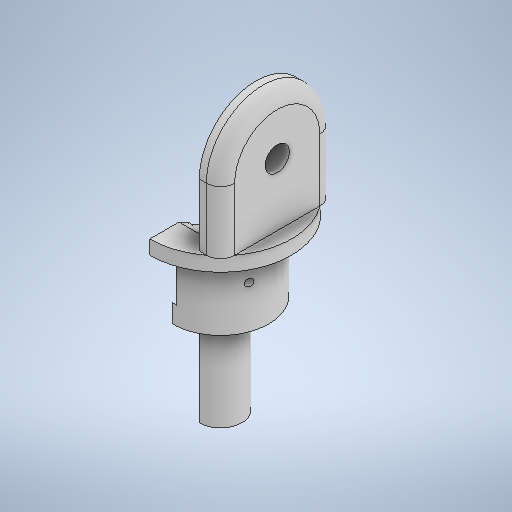
# Autodesk Inventor part: Haltevorrichtung1
Saved by Autodesk Inventor 2025 (Build 290162010, 162A)
## iProperties
Created: 2024-11-19
Part Number: Haltevorrichtung1
Material: Generisch
Document SubType Name: Modeling
Designer: jensb
Density: 1 g/cm^3
Appearance: Vorgabe
Author: jensb
Autodesk Inventor part; units mm, degrees
ref_plane "YZ Plane" through (0, 0, 0) normal (1, 0, 0) x (0, 1, 0)
ref_plane "XZ Plane" through (0, 0, 0) normal (0, 1, 0) x (-1, 0, 0)
ref_plane "XY Plane" through (0, 0, 0) normal (0, 0, 1) x (1, 0, 0)
sketch "Skizze1" plane through (0, 0, 0) normal (0, 0, 1) x (1, 0, 0)
  arc A0 (0, -15) -> (0, 15) centre (0, 0) ccw
  line L0 (0, -15) -> (0, 15)
  dimension "d27" = 15
  constraints: 2 end point, 2 point on circle, 1 centre point, 1 coincident, 1 vertical, 1 vertical alignment
  measures "d27" radius of A0
extrude "Extrusion1" add sketch "Skizze1" along normal blind 100
sketch "Skizze10" plane through (0, 0, 100) normal (0, 0, 1) x (1, 0, 0)
  arc A0 (0, -34) -> (0, 34) centre (0, 0) ccw
  line L0 (0, -34) -> (0, 34)
  dimension "d31" = 34
  constraints: 2 coincident, 2 end point, 2 point on circle, 1 centre point, 1 midpoint, 1 vertical
  measures "d31" radius of A0
extrude "Extrusion8" add sketch "Skizze10" along normal blind 20 and the other way blind 30
sketch "Skizze11" plane through (0, -15, 0) normal (-1, 0, 0) x (0, 0, 1)
  circle A0 centre (100, 3.2674) radius 25 construction
  circle A1 centre (174.0766, 15) radius 50 construction
  line L0 (174.0766, 15) -> (100, 15) construction
  line L1 (174.0766, 15) -> (100, 3.2674) construction
  circle A2 centre (100, 3.2674) radius 27.5 construction
  circle A3 centre (174.0766, 15) radius 52.5 construction
  line L2 (0, 30) -> (0, 0) construction
  line L3 (70, -19) -> (70, 0) construction
  circle A4 centre (174.0766, 15) radius 53
  point P0 (0, 15)
  point P1 (0, 15)
  dimension "d37" = 50
  dimension "d38" = 100
  dimension "d40" = 9
  dimension "d41" = 105
  dimension "d42" = 55
  dimension "d43" = 30
  dimension "d52" = 106
  dimension "d61" = 11.7326
  constraints: 5 centre point, 4 end point, 2 coincident, 1 horizontal, 1 horizontal alignment, 1 midpoint, 1 tangent, 1 vertical alignment
  measures "d37" diameter of A0
  measures "d38" diameter of A1
  measures "d40" angle of L0 L1
  measures "d41" diameter of A3
  measures "d42" diameter of A2
  measures "d43" distance from line of L3 L1.end
  measures "d52" diameter of A4
  measures "d61" distance from line of L0 L1.end
sketch "Skizze12" plane through (0, 0, 120) normal (0, 0, 1) x (1, 0, 0)
  arc A0 (0, -50) -> (0, 50) centre (0, 0) ccw
  line L0 (0, -50) -> (0, 50)
  dimension "d39" = 50
  constraints: 2 coincident, 2 end point, 2 point on circle, 1 centre point, 1 midpoint, 1 vertical
  measures "d39" radius of A0
extrude "Extrusion9" add sketch "Skizze12" along normal blind 10
sketch "Skizze9" plane through (0, -15, 0) normal (-1, 0, 0) x (0, 0, 1)
  circle A0 centre (100, 3.2674) radius 28
  line L0 (0, 30) -> (0, 0) projected
  circle A1 centre (100, 3.2674) radius 27.5 construction
  point P0 (0, 15)
  point P1 (100, 0)
  point P2 (0, 15)
  dimension "d28" = 56
  constraints: 1 centre point, 1 concentric, 1 midpoint
  measures "d28" diameter of A0
extrude "Extrusion7" cut sketch "Skizze9" against normal blind 2.5
sketch "Skizze13" plane through (0, -15, 0) normal (-1, 0, 0) x (0, 0, 1)
  line L0 (130, -35) -> (130, 65) projected
  line L1 (130, -25) -> (174.0766, -25)
  arc A0 (174.0766, -25) -> (174.0766, 55) centre (174.0766, 15) ccw
  line L2 (0, 30) -> (0, 0) projected
  line L3 (130, 55) -> (174.0766, 55)
  line L4 (-42.8153, 15) -> (256.892, 15) projected
  point P0 (0, 15)
  point P1 (0, 15)
  dimension "d46" = 80
  constraints: 4 end point, 2 point on circle, 2 point on line, 2 vertical alignment, 1 centre point, 1 coincident, 1 horizontal, 1 horizontal alignment, 1 midpoint, 1 tangent, 1 other
  measures "d46" diameter of A0
extrude "Extrusion10" add sketch "Skizze13" against normal blind 40
ref_plane "Arbeitsebene3" through (0, 0, 214.0766) normal (0, 0, 1) x (1, 0, 0)
sketch "Skizze14" plane through (0, 0, 214.0766) normal (0, 0, 1) x (1, 0, 0)
  line L0 (0, -40) -> (25, -40)
  line L1 (25, -40) -> (25, 40)
  line L2 (25, 40) -> (0, 40)
  line L3 (0, 40) -> (0, -40)
  line L4 (0, 40) -> (0, -40) projected
  point P0 (0, 0)
  point P1 (0, 0)
  dimension "d49" = 25
  dimension "d60" = 80
  constraints: 8 end point, 2 midpoint, 2 parallel, 1 coincident, 1 horizontal, 1 perpendicular
  measures "d49" distance of L0.start L0.end
  measures "d60" distance between parallel lines of L0 L2
extrude "Extrusion11" cut sketch "Skizze14" against normal up to surface (84.0766 mm away)
extrude "Extrusion12" cut sketch "Skizze11" against normal up to surface (25 mm away)
sketch "Skizze15" plane through (2.5, -15, 0) normal (-1, 0, 0) x (0, 0, 1)
  circle A0 centre (100, 3.2674) radius 2.5
  arc A1 (121.4484, 21.2665) -> (83.0247, -19) centre (100, 3.2674) ccw projected
  circle A2 centre (174.0766, 15) radius 8.5
  arc A3 (174.0766, -25) -> (174.0766, 55) centre (174.0766, 15) ccw projected
  point P0 (0, 15)
  dimension "d55" = 5
  dimension "d58" = 17
  constraints: 2 centre point, 2 concentric
  measures "d55" diameter of A0
  measures "d58" diameter of A2
extrude "Extrusion13" cut sketch "Skizze15" against normal through all
fillet "Rundung1" radius 10 3 edges at (40, 0, 214.0766) (40, -40, 152.0383) (40, 40, 152.0383)
